Autodesk Fusion 360 part; units mm, degrees
(part 2 of 2)
sketch "スケッチ21" plane through (0, -77, 0) normal (0, 1, 0) x (-1, 0, 0)
  line L0 (-144.5, 50) -> (-144.5, 53)
  line L1 (-144.5, 53) -> (-150, 53)
  line L2 (-150, 53) -> (-150, 56)
  line L3 (-150, 56) -> (-155.5, 56)
  line L4 (-155.5, 56) -> (-155.5, 59)
  line L5 (-155.5, 59) -> (-161, 59)
  line L6 (-161, 59) -> (-161, 62)
  line L7 (-161, 62) -> (-166.5, 62)
  line L8 (-166.5, 62) -> (-166.5, 65)
  line L9 (-166.5, 65) -> (-172, 65)
  line L10 (-172, 65) -> (-172, 68)
  line L11 (-172, 68) -> (-177.5, 68)
  line L12 (-177.5, 68) -> (-177.5, 71)
  line L13 (-177.5, 71) -> (-183, 71)
  line L14 (-183, 71) -> (-183, 74)
  line L15 (-183, 74) -> (-188.5, 74)
  line L16 (-188.5, 74) -> (-188.5, 77)
  line L17 (-188.5, 77) -> (-194, 77)
  line L18 (-194, 77) -> (-194, 80)
  line L19 (-194, 80) -> (-199.5, 80)
  line L20 (-199.5, 80) -> (-199.5, 3)
  arc A0 (-199.5, 3) -> (-196.5, 0) centre (-196.5, 3) ccw
  line L21 (-196.5, 0) -> (-3, 0)
  arc A1 (-3, 0) -> (0, 3) centre (-3, 3) ccw
  line L22 (0, 3) -> (0, 80)
  line L23 (0, 80) -> (-5.5, 80)
  line L24 (-5.5, 80) -> (-5.5, 77)
  line L25 (-5.5, 77) -> (-11, 77)
  line L26 (-11, 77) -> (-11, 74)
  line L27 (-11, 74) -> (-16.5, 74)
  line L28 (-16.5, 74) -> (-16.5, 71)
  line L29 (-16.5, 71) -> (-22, 71)
  line L30 (-22, 71) -> (-22, 68)
  line L31 (-22, 68) -> (-27.5, 68)
  line L32 (-27.5, 68) -> (-27.5, 65)
  line L33 (-27.5, 65) -> (-33, 65)
  line L34 (-33, 65) -> (-33, 62)
  line L35 (-33, 62) -> (-38.5, 62)
  line L36 (-38.5, 62) -> (-38.5, 59)
  line L37 (-38.5, 59) -> (-44, 59)
  line L38 (-44, 59) -> (-44, 56)
  line L39 (-44, 56) -> (-49.5, 56)
  line L40 (-49.5, 56) -> (-49.5, 53)
  line L41 (-49.5, 53) -> (-55, 53)
  line L42 (-55, 53) -> (-55, 50)
  line L43 (-55, 50) -> (-144.5, 50)
sketch "スケッチ22" plane through (0, -82.5, 0) normal (0, 1, 0) x (-1, 0, 0)
  line L0 (-150, 53) -> (-150, 56)
  line L1 (-150, 56) -> (-155.5, 56)
  line L2 (-155.5, 56) -> (-155.5, 59)
  line L3 (-155.5, 59) -> (-161, 59)
  line L4 (-161, 59) -> (-161, 62)
  line L5 (-161, 62) -> (-166.5, 62)
  line L6 (-166.5, 62) -> (-166.5, 65)
  line L7 (-166.5, 65) -> (-172, 65)
  line L8 (-172, 65) -> (-172, 68)
  line L9 (-172, 68) -> (-177.5, 68)
  line L10 (-177.5, 68) -> (-177.5, 71)
  line L11 (-177.5, 71) -> (-183, 71)
  line L12 (-183, 71) -> (-183, 74)
  line L13 (-183, 74) -> (-188.5, 74)
  line L14 (-188.5, 74) -> (-188.5, 77)
  line L15 (-188.5, 77) -> (-194, 77)
  line L16 (-194, 77) -> (-194, 80)
  line L17 (-194, 80) -> (-199.5, 80)
  line L18 (-199.5, 80) -> (-199.5, 3)
  arc A0 (-199.5, 3) -> (-196.5, 0) centre (-196.5, 3) ccw
  line L19 (-196.5, 0) -> (-3, 0)
  arc A1 (-3, 0) -> (0, 3) centre (-3, 3) ccw
  line L20 (0, 3) -> (0, 80)
  line L21 (0, 80) -> (-5.5, 80)
  line L22 (-5.5, 80) -> (-5.5, 77)
  line L23 (-5.5, 77) -> (-11, 77)
  line L24 (-11, 77) -> (-11, 74)
  line L25 (-11, 74) -> (-16.5, 74)
  line L26 (-16.5, 74) -> (-16.5, 71)
  line L27 (-16.5, 71) -> (-22, 71)
  line L28 (-22, 71) -> (-22, 68)
  line L29 (-22, 68) -> (-27.5, 68)
  line L30 (-27.5, 68) -> (-27.5, 65)
  line L31 (-27.5, 65) -> (-33, 65)
  line L32 (-33, 65) -> (-33, 62)
  line L33 (-33, 62) -> (-38.5, 62)
  line L34 (-38.5, 62) -> (-38.5, 59)
  line L35 (-38.5, 59) -> (-44, 59)
  line L36 (-44, 59) -> (-44, 56)
  line L37 (-44, 56) -> (-49.5, 56)
  line L38 (-49.5, 56) -> (-49.5, 53)
  line L39 (-49.5, 53) -> (-150, 53)
sketch "スケッチ23" plane through (0, -88, 0) normal (0, 1, 0) x (-1, 0, 0)
  line L0 (-155.5, 56) -> (-155.5, 59)
  line L1 (-155.5, 59) -> (-161, 59)
  line L2 (-161, 59) -> (-161, 62)
  line L3 (-161, 62) -> (-166.5, 62)
  line L4 (-166.5, 62) -> (-166.5, 65)
  line L5 (-166.5, 65) -> (-172, 65)
  line L6 (-172, 65) -> (-172, 68)
  line L7 (-172, 68) -> (-177.5, 68)
  line L8 (-177.5, 68) -> (-177.5, 71)
  line L9 (-177.5, 71) -> (-183, 71)
  line L10 (-183, 71) -> (-183, 74)
  line L11 (-183, 74) -> (-188.5, 74)
  line L12 (-188.5, 74) -> (-188.5, 77)
  line L13 (-188.5, 77) -> (-194, 77)
  line L14 (-194, 77) -> (-194, 80)
  line L15 (-194, 80) -> (-199.5, 80)
  line L16 (-199.5, 80) -> (-199.5, 3)
  arc A0 (-199.5, 3) -> (-196.5, 0) centre (-196.5, 3) ccw
  line L17 (-196.5, 0) -> (-3, 0)
  arc A1 (-3, 0) -> (0, 3) centre (-3, 3) ccw
  line L18 (0, 3) -> (0, 80)
  line L19 (0, 80) -> (-5.5, 80)
  line L20 (-5.5, 80) -> (-5.5, 77)
  line L21 (-5.5, 77) -> (-11, 77)
  line L22 (-11, 77) -> (-11, 74)
  line L23 (-11, 74) -> (-16.5, 74)
  line L24 (-16.5, 74) -> (-16.5, 71)
  line L25 (-16.5, 71) -> (-22, 71)
  line L26 (-22, 71) -> (-22, 68)
  line L27 (-22, 68) -> (-27.5, 68)
  line L28 (-27.5, 68) -> (-27.5, 65)
  line L29 (-27.5, 65) -> (-33, 65)
  line L30 (-33, 65) -> (-33, 62)
  line L31 (-33, 62) -> (-38.5, 62)
  line L32 (-38.5, 62) -> (-38.5, 59)
  line L33 (-38.5, 59) -> (-44, 59)
  line L34 (-44, 59) -> (-44, 56)
  line L35 (-44, 56) -> (-155.5, 56)
sketch "スケッチ24" plane through (0, -93.5, 0) normal (0, 1, 0) x (-1, 0, 0)
  line L0 (-161, 59) -> (-161, 62)
  line L1 (-161, 62) -> (-166.5, 62)
  line L2 (-166.5, 62) -> (-166.5, 65)
  line L3 (-166.5, 65) -> (-172, 65)
  line L4 (-172, 65) -> (-172, 68)
  line L5 (-172, 68) -> (-177.5, 68)
  line L6 (-177.5, 68) -> (-177.5, 71)
  line L7 (-177.5, 71) -> (-183, 71)
  line L8 (-183, 71) -> (-183, 74)
  line L9 (-183, 74) -> (-188.5, 74)
  line L10 (-188.5, 74) -> (-188.5, 77)
  line L11 (-188.5, 77) -> (-194, 77)
  line L12 (-194, 77) -> (-194, 80)
  line L13 (-194, 80) -> (-199.5, 80)
  line L14 (-199.5, 80) -> (-199.5, 3)
  arc A0 (-199.5, 3) -> (-196.5, 0) centre (-196.5, 3) ccw
  line L15 (-196.5, 0) -> (-3, 0)
  arc A1 (-3, 0) -> (0, 3) centre (-3, 3) ccw
  line L16 (0, 3) -> (0, 80)
  line L17 (0, 80) -> (-5.5, 80)
  line L18 (-5.5, 80) -> (-5.5, 77)
  line L19 (-5.5, 77) -> (-11, 77)
  line L20 (-11, 77) -> (-11, 74)
  line L21 (-11, 74) -> (-16.5, 74)
  line L22 (-16.5, 74) -> (-16.5, 71)
  line L23 (-16.5, 71) -> (-22, 71)
  line L24 (-22, 71) -> (-22, 68)
  line L25 (-22, 68) -> (-27.5, 68)
  line L26 (-27.5, 68) -> (-27.5, 65)
  line L27 (-27.5, 65) -> (-33, 65)
  line L28 (-33, 65) -> (-33, 62)
  line L29 (-33, 62) -> (-38.5, 62)
  line L30 (-38.5, 62) -> (-38.5, 59)
  line L31 (-38.5, 59) -> (-161, 59)
sketch "スケッチ25" plane through (0, -99, 0) normal (0, 1, 0) x (-1, 0, 0)
  line L0 (-166.5, 62) -> (-166.5, 65)
  line L1 (-166.5, 65) -> (-172, 65)
  line L2 (-172, 65) -> (-172, 68)
  line L3 (-172, 68) -> (-177.5, 68)
  line L4 (-177.5, 68) -> (-177.5, 71)
  line L5 (-177.5, 71) -> (-183, 71)
  line L6 (-183, 71) -> (-183, 74)
  line L7 (-183, 74) -> (-188.5, 74)
  line L8 (-188.5, 74) -> (-188.5, 77)
  line L9 (-188.5, 77) -> (-194, 77)
  line L10 (-194, 77) -> (-194, 80)
  line L11 (-194, 80) -> (-199.5, 80)
  line L12 (-199.5, 80) -> (-199.5, 3)
  arc A0 (-199.5, 3) -> (-196.5, 0) centre (-196.5, 3) ccw
  line L13 (-196.5, 0) -> (-3, 0)
  arc A1 (-3, 0) -> (0, 3) centre (-3, 3) ccw
  line L14 (0, 3) -> (0, 80)
  line L15 (0, 80) -> (-5.5, 80)
  line L16 (-5.5, 80) -> (-5.5, 77)
  line L17 (-5.5, 77) -> (-11, 77)
  line L18 (-11, 77) -> (-11, 74)
  line L19 (-11, 74) -> (-16.5, 74)
  line L20 (-16.5, 74) -> (-16.5, 71)
  line L21 (-16.5, 71) -> (-22, 71)
  line L22 (-22, 71) -> (-22, 68)
  line L23 (-22, 68) -> (-27.5, 68)
  line L24 (-27.5, 68) -> (-27.5, 65)
  line L25 (-27.5, 65) -> (-33, 65)
  line L26 (-33, 65) -> (-33, 62)
  line L27 (-33, 62) -> (-166.5, 62)
sketch "スケッチ26" plane through (0, -104.5, 0) normal (0, 1, 0) x (-1, 0, 0)
  line L0 (-172, 65) -> (-172, 68)
  line L1 (-172, 68) -> (-177.5, 68)
  line L2 (-177.5, 68) -> (-177.5, 71)
  line L3 (-177.5, 71) -> (-183, 71)
  line L4 (-183, 71) -> (-183, 74)
  line L5 (-183, 74) -> (-188.5, 74)
  line L6 (-188.5, 74) -> (-188.5, 77)
  line L7 (-188.5, 77) -> (-194, 77)
  line L8 (-194, 77) -> (-194, 80)
  line L9 (-194, 80) -> (-199.5, 80)
  line L10 (-199.5, 80) -> (-199.5, 3)
  arc A0 (-199.5, 3) -> (-196.5, 0) centre (-196.5, 3) ccw
  line L11 (-196.5, 0) -> (-3, 0)
  arc A1 (-3, 0) -> (0, 3) centre (-3, 3) ccw
  line L12 (0, 3) -> (0, 80)
  line L13 (0, 80) -> (-5.5, 80)
  line L14 (-5.5, 80) -> (-5.5, 77)
  line L15 (-5.5, 77) -> (-11, 77)
  line L16 (-11, 77) -> (-11, 74)
  line L17 (-11, 74) -> (-16.5, 74)
  line L18 (-16.5, 74) -> (-16.5, 71)
  line L19 (-16.5, 71) -> (-22, 71)
  line L20 (-22, 71) -> (-22, 68)
  line L21 (-22, 68) -> (-27.5, 68)
  line L22 (-27.5, 68) -> (-27.5, 65)
  line L23 (-27.5, 65) -> (-172, 65)
sketch "スケッチ27" plane through (0, -110, 0) normal (0, 1, 0) x (-1, 0, 0)
  line L0 (-16.5, 71) -> (-22, 71)
  line L1 (-22, 71) -> (-22, 68)
  line L2 (-22, 68) -> (-177.5, 68)
  line L3 (-177.5, 68) -> (-177.5, 71)
  line L4 (-177.5, 71) -> (-183, 71)
  line L5 (-183, 71) -> (-183, 74)
  line L6 (-183, 74) -> (-188.5, 74)
  line L7 (-188.5, 74) -> (-188.5, 77)
  line L8 (-188.5, 77) -> (-194, 77)
  line L9 (-194, 77) -> (-194, 80)
  line L10 (-194, 80) -> (-199.5, 80)
  line L11 (-199.5, 80) -> (-199.5, 3)
  arc A0 (-199.5, 3) -> (-196.5, 0) centre (-196.5, 3) ccw
  line L12 (-196.5, 0) -> (-3, 0)
  arc A1 (-3, 0) -> (0, 3) centre (-3, 3) ccw
  line L13 (0, 3) -> (0, 80)
  line L14 (0, 80) -> (-5.5, 80)
  line L15 (-5.5, 80) -> (-5.5, 77)
  line L16 (-5.5, 77) -> (-11, 77)
  line L17 (-11, 77) -> (-11, 74)
  line L18 (-11, 74) -> (-16.5, 74)
  line L19 (-16.5, 74) -> (-16.5, 71)
sketch "スケッチ28" plane through (0, -115.5, 0) normal (0, 1, 0) x (-1, 0, 0)
  line L0 (-183, 71) -> (-183, 74)
  line L1 (-183, 74) -> (-188.5, 74)
  line L2 (-188.5, 74) -> (-188.5, 77)
  line L3 (-188.5, 77) -> (-194, 77)
  line L4 (-194, 77) -> (-194, 80)
  line L5 (-194, 80) -> (-199.5, 80)
  line L6 (-199.5, 80) -> (-199.5, 3)
  arc A0 (-199.5, 3) -> (-196.5, 0) centre (-196.5, 3) ccw
  line L7 (-196.5, 0) -> (-3, 0)
  arc A1 (-3, 0) -> (0, 3) centre (-3, 3) ccw
  line L8 (0, 3) -> (0, 80)
  line L9 (0, 80) -> (-5.5, 80)
  line L10 (-5.5, 80) -> (-5.5, 77)
  line L11 (-5.5, 77) -> (-11, 77)
  line L12 (-11, 77) -> (-11, 74)
  line L13 (-11, 74) -> (-16.5, 74)
  line L14 (-16.5, 74) -> (-16.5, 71)
  line L15 (-16.5, 71) -> (-183, 71)
sketch "スケッチ29" plane through (0, -121, 0) normal (0, 1, 0) x (-1, 0, 0)
  line L0 (-188.5, 74) -> (-188.5, 77)
  line L1 (-188.5, 77) -> (-194, 77)
  line L2 (-194, 77) -> (-194, 80)
  line L3 (-194, 80) -> (-199.5, 80)
  line L4 (-199.5, 80) -> (-199.5, 3)
  arc A0 (-199.5, 3) -> (-196.5, 0) centre (-196.5, 3) ccw
  line L5 (-196.5, 0) -> (-3, 0)
  arc A1 (-3, 0) -> (0, 3) centre (-3, 3) ccw
  line L6 (0, 3) -> (0, 80)
  line L7 (0, 80) -> (-5.5, 80)
  line L8 (-5.5, 80) -> (-5.5, 77)
  line L9 (-5.5, 77) -> (-11, 77)
  line L10 (-11, 77) -> (-11, 74)
  line L11 (-11, 74) -> (-188.5, 74)
sketch "スケッチ30" plane through (0, -126.5, 0) normal (0, 1, 0) x (-1, 0, 0)
  line L0 (-194, 77) -> (-194, 80)
  line L1 (-194, 80) -> (-199.5, 80)
  line L2 (-199.5, 80) -> (-199.5, 3)
  arc A0 (-199.5, 3) -> (-196.5, 0) centre (-196.5, 3) ccw
  line L3 (-196.5, 0) -> (-3, 0)
  arc A1 (-3, 0) -> (0, 3) centre (-3, 3) ccw
  line L4 (0, 3) -> (0, 80)
  line L5 (0, 80) -> (-5.5, 80)
  line L6 (-5.5, 80) -> (-5.5, 77)
  line L7 (-5.5, 77) -> (-194, 77)
sketch "スケッチ31" plane through (0, -132, 0) normal (0, 1, 0) x (-1, 0, 0)
  line L0 (-196.5, 0) -> (-3, 0)
  arc A0 (-3, 0) -> (0, 3) centre (-3, 3) ccw
  line L1 (0, 3) -> (0, 80)
  line L2 (0, 80) -> (-199.5, 80)
  line L3 (-199.5, 80) -> (-199.5, 3)
  arc A1 (-199.5, 3) -> (-196.5, 0) centre (-196.5, 3) ccw
sketch "スケッチ32" plane through (0, 0, 88) normal (0, 0, 1) x (-1, 0, 0)
  line L0 (-183.5, 45.25) -> (-183.5, 92.25)
  line L1 (-183.5, 92.25) -> (-141, 92.25)
  line L2 (-141, 92.25) -> (-141, 45.25)
  line L3 (-141, 45.25) -> (-183.5, 45.25)
  line L4 (-78.5, 45.25) -> (-121, 45.25)
  line L5 (-121, 45.25) -> (-121, 92.25)
  line L6 (-121, 92.25) -> (-78.5, 92.25)
  line L7 (-78.5, 92.25) -> (-78.5, 45.25)
  line L8 (-58.5, 92.25) -> (-16, 92.25)
  line L9 (-16, 92.25) -> (-16, 45.25)
  line L10 (-16, 45.25) -> (-58.5, 45.25)
  line L11 (-58.5, 45.25) -> (-58.5, 92.25)
  line L12 (-199.5, 0) -> (0, 0)
  line L13 (0, 0) -> (0, 137.5)
  line L14 (0, 137.5) -> (-199.5, 137.5)
  line L15 (-199.5, 137.5) -> (-199.5, 0)
sketch "スケッチ33" plane through (0, 0, 84) normal (0, 0, 1) x (-1, 0, 0)
  line L0 (-199.5, 0) -> (0, 0)
  line L1 (0, 0) -> (0, 137.5)
  line L2 (0, 137.5) -> (-199.5, 137.5)
  line L3 (-199.5, 137.5) -> (-199.5, 0)
